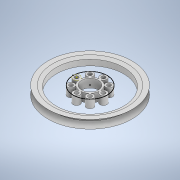
# Autodesk Inventor part: Spool1
Saved by Autodesk Inventor 2021 (Build 250183000, 183)
## iProperties
Created: 2022-08-29
Part Number: Spool1
Material: Generic
Document SubType Name: Modeling
Designer: alyn649
Density: 1 g/cm^3
Appearance: Default
Author: alyn649
Autodesk Inventor part; units mm, degrees
ref_plane "YZ Plane" through (0, 0, 0) normal (1, 0, 0) x (0, 1, 0)
ref_plane "XZ Plane" through (0, 0, 0) normal (0, 1, 0) x (-1, 0, 0)
ref_plane "XY Plane" through (0, 0, 0) normal (0, 0, 1) x (1, 0, 0)
sketch "Sketch1" plane through (0, 0, 0) normal (0, 1, 0) x (-1, 0, 0)
  circle A0 centre (0, 0) radius 25
  circle A1 centre (0, 0) radius 8 construction
  circle A2 centre (0, -8) radius 1.1
  circle A3 centre (5.6569, -5.6569) radius 1.1
  circle A4 centre (8, 0) radius 1.1
  circle A5 centre (5.6569, 5.6569) radius 1.1
  circle A6 centre (0, 8) radius 1.1
  circle A7 centre (-5.6569, 5.6569) radius 1.1
  circle A8 centre (-8, 0) radius 1.1
  circle A9 centre (-5.6569, -5.6569) radius 1.1
  dimension "d1" = 16
  dimension "d0" = 50
  dimension "d2" = 2.2
  dimension "d6" = 360
  constraints: 9 centre point, 2 coincident, 2 vertical alignment, 19 other
  measures "d0" diameter of A0
  measures "d2" diameter of A2
extrude "Extrusion1" add sketch "Sketch1" along normal blind 5
sketch "Sketch2" plane through (0, 5, 0) normal (0, 1, 0) x (1, 0, 0)
  circle A0 centre (0, 0) radius 5
  dimension "d10" = 10
  constraints: 1 centre point, 1 coincident
  measures "d10" diameter of A0
extrude "Extrusion2" cut sketch "Sketch2" against normal blind 5
sketch "Sketch3" plane through (0, 0, 0) normal (0, 0, 1) x (1, 0, 0)
  line L0 (25, 5) -> (-25, 5) projected
  line L1 (25, 0) -> (-25, 0) projected
  line L2 (-25, 5) -> (-21, 3.5)
  line L3 (-21, 3.5) -> (-21, 1.5)
  line L4 (-25, 0) -> (-25, 5) projected
  line L5 (25, 0) -> (-25, 0) projected
  line L6 (-21, 1.5) -> (-25, 0)
  line L7 (0, -1) -> (0, 6) projected
  point P0 (0, 0)
  point P1 (-21, 2.5)
  point P2 (-25, 2.5)
  dimension "d13" = 2
  dimension "d14" = 4
  constraints: 6 end point, 2 midpoint, 1 horizontal alignment, 1 parallel
  measures "d13" distance of L2.end L3.end
  measures "d14" distance between parallel lines of L4 L3
revolve "Revolution1" cut sketch "Sketch3" angle 360 about axis through (0, -10, 0) along (0, 1, 0) contours L2 L3 L6 L4
shell "Shell1" thickness 1 removed faces 2 at (-18.4111, 5, 6.1101) at (-18.4111, 0, 6.1101)
sketch "Sketch4" plane through (0, 5, 0) normal (0, 1, 0) x (1, 0, 0)
  circle A0 centre (0, 0) radius 10.1
  arc A1 (-5.9744, 0.5539) -> (-5.9744, -0.5539) centre (-8, 0) ccw construction
  point P0 (-10.1, 0)
  constraints: 1 coincident, 1 horizontal alignment, 1 point on circle, 2 other
body "Solid1"
